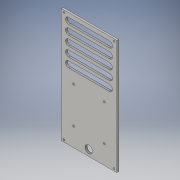
# Autodesk Inventor part: RaspberryBox_Backplate
Saved by Autodesk Inventor 2016 (Build 200138000, 138)
## iProperties
Created: 2016-12-27
Part Number: RaspberryBox_Backplate
Material: Generisch
Document SubType Name: Modeling
Designer: Moritz
Density: 1 g/cm^3
Appearance: Vorgabe
Author: Moritz
Autodesk Inventor part; units mm, degrees
ref_plane "YZ Plane" through (0, 0, 0) normal (1, 0, 0) x (0, 1, 0)
ref_plane "XZ Plane" through (0, 0, 0) normal (0, 1, 0) x (-1, 0, 0)
ref_plane "XY Plane" through (0, 0, 0) normal (0, 0, 1) x (1, 0, 0)
sketch "Skizze1" plane through (0, 0, 0) normal (0, 1, 0) x (-1, 0, 0)
  line L0 (-44.3, 91.3) -> (44.3, 91.3)
  line L1 (44.3, 91.3) -> (44.3, -91.3)
  line L2 (44.3, -91.3) -> (-44.3, -91.3)
  line L3 (-44.3, -91.3) -> (-44.3, 91.3)
  line L4 (-44.3, 91.3) -> (44.3, -91.3) construction
  line L5 (44.3, 91.3) -> (-44.3, -91.3) construction
  point P0 (0, 0)
  dimension "d0" = 88.6
  dimension "d1" = 182.6
  constraints: 12 end point, 2 midpoint, 2 parallel, 1 horizontal, 1 perpendicular
  measures "d0" distance of L1.end L2.end
  measures "d1" distance of L0.end L1.end
extrude "Extrusion1" add sketch "Skizze1" along normal blind 3
sketch "Skizze2" plane through (0, 0, 0) normal (0, -1, 0) x (1, 0, 0)
  line L0 (-44.3, -91.3) -> (44.3, -91.3) projected
  line L1 (0, -91.3) -> (0, 91.3)
  line L2 (44.3, 91.3) -> (-44.3, 91.3) projected
  line L3 (-24.5, -61.3) -> (24.5, -61.3)
  line L4 (24.5, -61.3) -> (24.5, -3.3)
  line L5 (24.5, -3.3) -> (-24.5, -3.3)
  line L6 (-24.5, -3.3) -> (-24.5, -61.3)
  line L7 (-24.5, -61.3) -> (24.5, -3.3) construction
  line L8 (24.5, -61.3) -> (-24.5, -3.3) construction
  point P0 (0, 0)
  point P1 (0, -32.3)
  dimension "d5" = 49
  dimension "d6" = 58
  dimension "d7" = 30
  constraints: 14 end point, 4 midpoint, 2 parallel, 1 horizontal, 1 perpendicular, 1 point on line
  measures "d5" distance of L5.end L4.end
  measures "d6" distance of L4.end L3.end
  measures "d7" distance between parallel lines of L0 L3
hole "Bohrung1" at (-24.5, 0, -61.3) at (24.5, 0, -61.3) at (24.5, 0, -3.3) at (-24.5, 0, -3.3) direction (0, 1, 0) diameter 3 depth 2.5
sketch "Skizze3" plane through (0, 0, 0) normal (0, -1, 0) x (1, 0, 0)
  line L0 (32.5, 15.0873) -> (-32.5, 15.0873)
  line L1 (-37.5, 20.0873) -> (-37.5, 20.0873)
  line L2 (-32.5, 25.0873) -> (32.5, 25.0873)
  line L3 (37.5, 20.0873) -> (37.5, 20.0873)
  line L4 (37.5, 15.0873) -> (-37.5, 25.0873) construction
  line L5 (-37.5, 15.0873) -> (37.5, 25.0873) construction
  arc A0 (-37.5, 20.0873) -> (-32.5, 15.0873) centre (-32.5, 20.0873) ccw
  arc A1 (-32.5, 25.0873) -> (-37.5, 20.0873) centre (-32.5, 20.0873) ccw
  arc A2 (32.5, 15.0873) -> (37.5, 20.0873) centre (32.5, 20.0873) ccw
  arc A3 (37.5, 20.0873) -> (32.5, 25.0873) centre (32.5, 20.0873) ccw
  point P0 (0, 0)
  point P1 (0, 20.0873)
  dimension "d15" = 75
  dimension "d16" = 10
  dimension "d18" = 5
  dimension "d19" = 5
  dimension "d20" = 5
  constraints: 12 end point, 8 point on circle, 8 point on line, 8 tangent, 4 centre point, 2 midpoint, 2 parallel, 1 concentric, 1 horizontal, 1 perpendicular
  measures "d15" distance of L4.end L5.end
  measures "d16" distance of L5.start L4.end
  measures "d18" radius of A0
  measures "d19" radius of A2
  measures "d20" radius of A3
extrude "Extrusion2" cut sketch "Skizze3" against normal blind 10
pattern_linear "Rechteckige Anordnung1" count 5 spacing 15 along (0, 0, 1) of "Extrusion2"
hole "Bohrung2" at (-39.9, 0, -87.9) direction (0, 1, 0) diameter 3 depth 8 tip angle 118
mirror "Spiegeln1" about plane through (0, 0, 0) normal (1, 0, 0) of "Bohrung2"
mirror "Spiegeln2" about plane through (0, 0, 0) normal (0, 0, 1) of "Bohrung2", "Spiegeln1"
hole "Bohrung3" at (-0.3, 0, -81.3) direction (0, 1, 0) diameter 11.8 depth 8 tip angle 118
